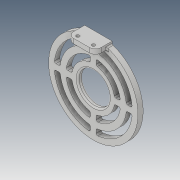
# Autodesk Inventor part: backSideThrusterCover
Saved by Autodesk Inventor 2018 (Build 220112000, 112)
## iProperties
Created: 2020-02-23
Part Number: backSideThrusterCover
Material: Generic
Document SubType Name: Modeling
Designer: anirudh
Density: 1 g/cm^3
Appearance: Default
Author: anirudh
Autodesk Inventor part; units mm, degrees
ref_plane "YZ Plane" through (0, 0, 0) normal (1, 0, 0) x (0, 1, 0)
ref_plane "XZ Plane" through (0, 0, 0) normal (0, 1, 0) x (-1, 0, 0)
ref_plane "XY Plane" through (0, 0, 0) normal (0, 0, 1) x (1, 0, 0)
sketch "Sketch1" plane through (0, 0, 0) normal (0, 0, 1) x (1, 0, 0)
  line L0 (3, 0) -> (-3, 0)
  line L1 (0, 0) -> (13.85, 0)
  line L2 (14.85, -3.0647) -> (14.85, -1)
  line L3 (14.85, -3.0647) -> (14.85, -1)
  line L4 (0, 0) -> (-13.85, 0)
  line L5 (13.85, 0) -> (-13.85, 0)
  line L6 (-14.85, -3.0647) -> (-14.85, -1)
  line L7 (-14.85, -3.0647) -> (-14.85, -1)
  arc A0 (47.8846, -42.8653) -> (14.85, -3.0647) centre (0, -49) ccw
  arc A1 (-14.85, -3.0647) -> (14.85, -3.0647) centre (0, -49) ccw
  line L8 (-14.85, -1) -> (-14.85, 0)
  line L9 (-14.85, 0) -> (-13.85, 0)
  line L10 (14.85, -1) -> (14.85, 0)
  line L11 (14.85, 0) -> (13.85, 0)
  circle A2 centre (0, -49) radius 16.8275
  line L12 (-3.175, -26.041) -> (-3.175, -19.6437)
  line L13 (-3.175, -13.2633) -> (-3.175, -6.892)
  line L14 (3.175, -26.041) -> (3.175, -19.6437)
  line L15 (3.175, -13.2633) -> (3.175, -6.892)
  arc A3 (-3.175, -26.041) -> (-22.959, -45.825) centre (0, -49) ccw
  arc A4 (-3.175, -19.6437) -> (-29.3563, -45.825) centre (0, -49) ccw
  line L16 (-22.959, -45.825) -> (-29.3563, -45.825)
  line L17 (-35.7367, -45.825) -> (-42.108, -45.825)
  line L18 (-22.959, -52.175) -> (-29.3563, -52.175)
  line L19 (-35.7367, -52.175) -> (-42.108, -52.175)
  arc A5 (-3.175, -13.2633) -> (-35.7367, -45.825) centre (0, -49) ccw
  arc A6 (-3.175, -6.892) -> (-42.108, -45.825) centre (0, -49) ccw
  arc A7 (-22.959, -52.175) -> (-3.175, -71.959) centre (0, -49) ccw
  arc A8 (-29.3563, -52.175) -> (-3.175, -78.3563) centre (0, -49) ccw
  line L20 (-3.175, -71.959) -> (-3.175, -78.3563)
  line L21 (-3.175, -84.7367) -> (-3.175, -91.108)
  line L22 (3.175, -71.959) -> (3.175, -78.3563)
  line L23 (3.175, -84.7367) -> (3.175, -91.108)
  arc A9 (-35.7367, -52.175) -> (-3.175, -84.7367) centre (0, -49) ccw
  arc A10 (-42.108, -52.175) -> (-3.175, -91.108) centre (0, -49) ccw
  arc A11 (3.175, -71.959) -> (22.959, -52.175) centre (0, -49) ccw
  arc A12 (22.959, -45.825) -> (3.175, -26.041) centre (0, -49) ccw
  arc A13 (3.175, -78.3563) -> (29.3563, -52.175) centre (0, -49) ccw
  arc A14 (29.3563, -45.825) -> (3.175, -19.6437) centre (0, -49) ccw
  line L24 (22.959, -45.825) -> (29.3563, -45.825)
  line L25 (35.7367, -45.825) -> (42.108, -45.825)
  line L26 (22.959, -52.175) -> (29.3563, -52.175)
  line L27 (35.7367, -52.175) -> (42.108, -52.175)
  arc A15 (3.175, -84.7367) -> (35.7367, -52.175) centre (0, -49) ccw
  arc A16 (35.7367, -45.825) -> (3.175, -13.2633) centre (0, -49) ccw
  arc A17 (3.175, -91.108) -> (42.108, -52.175) centre (0, -49) ccw
  arc A18 (42.108, -45.825) -> (3.175, -6.892) centre (0, -49) ccw
  point P0 (0, 0)
  point P1 (-16.85, -4.0995)
  constraints: 57 end point, 36 point on circle, 19 centre point, 8 parallel, 6 coincident, 6 perpendicular, 5 vertical, 2 horizontal, 1 collinear, 1 midpoint
ref_plane "Work Plane1" through (0, 0, 5.588) normal (0, 0, 1) x (1, 0, 0)
sketch "Sketch3" plane through (0, 0, 5.588) normal (0, 0, 1) x (1, 0, 0)
  line L0 (14.85, 0) -> (-14.85, 0) projected
  line L1 (-14.85, 0) -> (14.85, 0)
  line L2 (14.85, 0) -> (14.85, -5.08)
  line L3 (14.85, -5.08) -> (-14.85, -5.08)
  line L4 (-14.85, -5.08) -> (-14.85, 0)
  point P0 (0, 0)
  dimension "d16" = 5.08
  constraints: 8 end point, 2 parallel, 1 horizontal, 1 perpendicular
  measures "d16" distance of L1.end L2.end
extrude "Extrusion2" add sketch "Sketch3" along normal blind 12.7
ref_plane "Work Plane2" through (-8.5, -5.08, 18.288) normal (0, -1, 0) x (1, 0, 0)
sketch "Sketch4" plane through (-8.5, -5.08, 18.288) normal (0, -1, 0) x (1, 0, 0)
  line L0 (17, 0) -> (0, 0) projected
  circle A0 centre (0, -4.445) radius 1.75
  circle A1 centre (17, -4.445) radius 1.75
  point P0 (8.5, -18.288)
  dimension "d22" = 3.5
  dimension "d23" = 3.5
  constraints: 2 centre point
  measures "d22" diameter of A0
  measures "d23" diameter of A1
extrude "Extrusion3" cut sketch "Sketch4" against normal blind 10.16
extrude "Extrusion4" add sketch "Sketch1" along normal blind 5.588
fillet "Fillet5" radius 6.35 2 edges at (-14.85, -2.54, 18.288) (14.85, -2.54, 18.288)
fillet "Fillet6" radius 1.5875 5 edges at (0, -5.08, 5.588) (14.85, -3.0647, 2.794) (14.85, -4.0724, 5.588) (-14.85, -3.0647, 2.794) (-14.85, -4.0724, 5.588)
fillet "Fillet7" radius 1.5875 34 edges at (-3.175, -6.892, 2.794) (-3.175, -13.2633, 2.794) (-3.175, -19.6437, 2.794) (-3.175, -26.041, 2.794) (-42.108, -45.825, 2.794) (-35.7367, -45.825, 2.794) (-29.3563, -45.825, 2.794) (-22.959, -45.825, 2.794) (-42.108, -52.175, 2.794) (-35.7367, -52.175, 2.794) (-29.3563, -52.175, 2.794) (-22.959, -52.175, 2.794) (-3.175, -71.959, 2.794) (-3.175, -78.3563, 2.794) (-3.175, -84.7367, 2.794) (-3.175, -91.108, 2.794) (3.175, -91.108, 2.794) (3.175, -84.7367, 2.794) (3.175, -78.3563, 2.794) (3.175, -71.959, 2.794) (22.959, -52.175, 2.794) (29.3563, -52.175, 2.794) (35.7367, -52.175, 2.794) (42.108, -52.175, 2.794) (42.108, -45.825, 2.794) (35.7367, -45.825, 2.794) (29.3563, -45.825, 2.794) (22.959, -45.825, 2.794) (3.175, -26.041, 2.794) (3.175, -19.6437, 2.794) (3.175, -13.2633, 2.794) (3.175, -6.892, 2.794) (-16.8275, -49, 0) (-16.8275, -49, 5.588)
body "Solid1"
